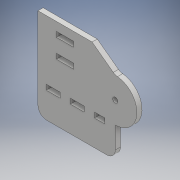
# Autodesk Inventor part: codo2
Saved by Autodesk Inventor 2018 (Build 220112000, 112)
## iProperties
Created: 2020-03-10
Part Number: codo2
Material: Genérico
Document SubType Name: Modeling
Designer: sala.ceri
Density: 1 g/cm^3
Appearance: Valor por defecto
Author: sala.ceri
Autodesk Inventor part; units mm, degrees
ref_plane "YZ Plane" through (0, 0, 0) normal (1, 0, 0) x (0, 1, 0)
ref_plane "XZ Plane" through (0, 0, 0) normal (0, 1, 0) x (-1, 0, 0)
ref_plane "XY Plane" through (0, 0, 0) normal (0, 0, 1) x (1, 0, 0)
sketch "Boceto1" plane through (0, 0, 0) normal (0, 1, 0) x (-1, 0, 0)
  arc A0 (117.4998, -25.6738) -> (124.3299, -32.5039) centre (119.9998, -30.0039) ccw
  circle A1 centre (119.9998, -30.0039) radius 1.5
  line L0 (119.9998, -12.5039) -> (119.9998, -21.3437)
  arc A2 (117.4998, -25.6738) -> (119.9998, -21.3437) centre (114.9998, -21.3437) ccw
  arc A3 (128.66, -30.0039) -> (124.3299, -32.5039) centre (128.66, -35.0039) ccw
  arc A4 (118.7343, 12.4319) -> (119.9998, -12.5039) centre (119.9994, -0.0039) ccw
  line L1 (133.4998, 22.4961) -> (121.2045, 13.3885)
  line L2 (164.9248, 22.4961) -> (164.9248, -25.0039)
  line L3 (159.9248, -30.0039) -> (128.66, -30.0039)
  line L4 (164.9248, 22.4961) -> (133.4998, 22.4961)
  line L5 (149.2123, 17.4961) -> (144.2123, 17.4961)
  line L6 (144.2123, 17.4961) -> (144.2123, 14.4961)
  line L7 (144.2123, 14.4961) -> (154.2123, 14.4961)
  line L8 (154.2123, 14.4961) -> (154.2123, 17.4961)
  line L9 (154.2123, 17.4961) -> (149.2123, 17.4961)
  line L10 (149.2123, 6.4961) -> (144.2123, 6.4961)
  line L11 (144.2123, 6.4961) -> (144.2123, 3.4961)
  line L12 (144.2123, 3.4961) -> (154.2123, 3.4961)
  line L13 (154.2123, 3.4961) -> (154.2123, 6.4961)
  line L14 (154.2123, 6.4961) -> (149.2123, 6.4961)
  line L15 (160.0685, -12.0039) -> (160.0685, -15.0039)
  circle A5 centre (119.9994, -0.0039) radius 1.5
  line L16 (160.0685, -12.0039) -> (152.0685, -12.0039)
  line L17 (152.0685, -12.0039) -> (152.0685, -15.0039)
  line L18 (152.0685, -15.0039) -> (160.0685, -15.0039)
  line L19 (146.0685, -12.0039) -> (146.0685, -15.0039)
  line L20 (146.0685, -15.0039) -> (138.0685, -15.0039)
  line L21 (138.0685, -15.0039) -> (138.0685, -12.0039)
  line L22 (132.0685, -12.0039) -> (132.0685, -15.0039)
  line L23 (132.0685, -15.0039) -> (126.0685, -15.0039)
  line L24 (126.0685, -15.0039) -> (126.0685, -12.0039)
  line L25 (126.0685, -12.0039) -> (132.0685, -12.0039)
  line L26 (138.0685, -12.0039) -> (146.0685, -12.0039)
  arc A6 (159.9248, -30.0039) -> (164.9248, -25.0039) centre (159.9248, -25.0039) ccw
  arc A7 (118.7343, 12.4319) -> (121.2045, 13.3885) centre (118.2283, 17.4062) ccw
  point P0 (124.9998, -30.0039)
  point P1 (119.9998, -25.0039)
  point P2 (119.9998, 12.4961)
  dimension "d165" = 8
  dimension "d166" = 6
  dimension "d167" = 8
  dimension "d169" = 6
  dimension "d170" = 5
  constraints: 54 end point, 15 point on circle, 14 perpendicular, 8 centre point, 7 point on line, 7 tangent, 4 vertical, 2 coincident, 1 equal radius, 1 horizontal
  measures "d165" distance of L15.start L16.end
  measures "d166" distance of L16.end L19.start
  measures "d167" distance of L19.end L20.end
  measures "d169" distance of L22.end L23.end
  measures "d170" radius of A6
extrude "Extrusión1" add sketch "Boceto1" along normal blind 3
sketch "Boceto2" plane through (0, 0, 0) normal (0, -1, 0) x (1, 0, 0)
  line L0 (-128.66, -30.0039) -> (-159.9248, -30.0039) projected
  line L1 (-128.66, -30.0039) -> (-124.9998, -30.0039)
  line L2 (-119.9998, -25.0039) -> (-119.9998, -21.3437)
  line L3 (-119.9998, -21.3437) -> (-111.1429, -30.5208)
  line L4 (-111.1429, -30.5208) -> (-116.7612, -39.5335)
  line L5 (-116.7612, -39.5335) -> (-128.66, -30.0039)
  arc A0 (-124.9998, -30.0039) -> (-119.9998, -25.0039) centre (-124.9998, -25.0039) ccw
  point P0 (0, 0)
  point P1 (-119.9998, -30.0039)
  constraints: 10 end point, 2 point on circle, 2 point on line, 2 tangent, 1 centre point, 1 horizontal, 1 perpendicular
extrude "Extrusión2" cut sketch "Boceto2" against normal blind 10
